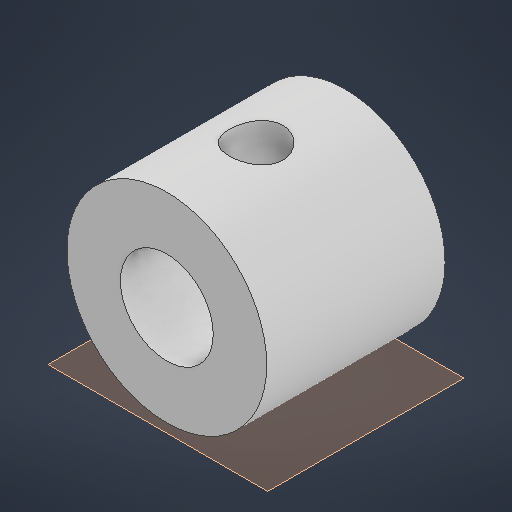
# Autodesk Inventor part: Differential_drive_lock
Saved by Autodesk Inventor 2026 (Build 300175000, 175)
## iProperties
Created: 2025-07-10
Part Number: Differential_drive_lock
Material: Generic
Document SubType Name: Modeling
Designer: user
Density: 1 g/cm^3
Appearance: Default
Author: user
Autodesk Inventor part; units mm, degrees
ref_plane "YZ Plane" through (0, 0, 0) normal (1, 0, 0) x (0, 1, 0)
ref_plane "XY Plane" through (0, 0, 0) normal (0, 0, 1) x (1, 0, 0)
sketch "Sketch1" plane through (0, 0, 0) normal (0, 0, 1) x (1, 0, 0)
  circle A0 centre (0, 0) radius 2.6
  circle A1 centre (0, 0) radius 5.6
  dimension "d0" = 5.2
  dimension "d1" = 3
  constraints: 2 centre point, 1 coincident
  measures "d0" diameter of A0
  measures "d1" radial gap between concentric circles of A0 A1
extrude "Extrusion1" add sketch "Sketch1" along normal blind 10
ref_plane "Work Plane1" through (0, -5.6, 0) normal (0, 1, 0) x (-1, 0, 0)
sketch "Sketch2" plane through (0, -5.6, 0) normal (0, 1, 0) x (-1, 0, 0)
  circle A0 centre (0, 5) radius 1.5
  line L0 (5.6, 10) -> (-5.6, 10) projected
  point P0 (0, 0)
  dimension "d4" = 3
  dimension "d5" = 5
  constraints: 1 centre point
  measures "d4" diameter of A0
  measures "d5" distance from line of L0 A0.centre
extrude "Extrusion2" cut sketch "Sketch2" along normal through all
body "Solid1"
